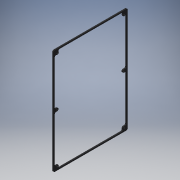
# Autodesk Inventor part: gasket
Saved by Autodesk Inventor 2019 (Build 230136000, 136)
## iProperties
Created: 2020-02-21
Part Number: gasket
Material: Generic
Document SubType Name: Modeling
Designer: ntb11189
Density: 1 g/cm^3
Appearance: Rubber - Black
Author: ntb11189
Autodesk Inventor part; units mm, degrees
ref_plane "YZ Plane" through (0, 0, 0) normal (1, 0, 0) x (0, 1, 0)
ref_plane "XZ Plane" through (0, 0, 0) normal (0, 1, 0) x (-1, 0, 0)
ref_plane "XY Plane" through (0, 0, 0) normal (0, 0, 1) x (1, 0, 0)
sketch "Sketch1" plane through (0, 0, 0) normal (1, 0, 0) x (0, 1, 0)
  line L0 (-4.25, -58.4) -> (-75.9, -58.4)
  arc A0 (-78.2159, -55.4407) -> (-75.9, -58.4) centre (-75.9, -56.0141) ccw
  arc A1 (-78.2159, -55.4407) -> (-80.9407, -52.7159) centre (-80.4, -54.9) ccw
  arc A2 (-83.9, -50.4) -> (-80.9407, -52.7159) centre (-81.5141, -50.4) ccw
  line L1 (-83.9, -50.4) -> (-83.9, 50.4)
  arc A3 (-81.3323, 52.0522) -> (-83.9, 50.4) centre (-82.0846, 50.4) ccw
  arc A4 (-81.3323, 52.0522) -> (-78.2997, 54.9071) centre (-80.4, 54.1) ccw
  arc A5 (-75.9, 58.4) -> (-78.2997, 54.9071) centre (-75.9, 55.8292) ccw
  line L2 (-75.9, 58.4) -> (-4.25, 58.4)
  arc A6 (-2.25, 56.4) -> (-4.25, 58.4) centre (-4.25, 56.4) ccw
  line L3 (-2.25, 56.4) -> (-2.25, 54.5)
  arc A7 (-2.25, 54.5) -> (2.25, 54.5) centre (0, 54.5) ccw
  line L4 (2.25, 54.5) -> (2.25, 56.4)
  arc A8 (4.25, 58.4) -> (2.25, 56.4) centre (4.25, 56.4) ccw
  line L5 (4.25, 58.4) -> (75.9, 58.4)
  arc A9 (77.6729, 55.2614) -> (75.9, 58.4) centre (75.9, 56.33) ccw
  arc A10 (77.6729, 55.2614) -> (80.7614, 52.1729) centre (79.6, 54.1) ccw
  arc A11 (83.9, 50.4) -> (80.7614, 52.1729) centre (81.83, 50.4) ccw
  line L6 (83.9, 50.4) -> (83.9, -50.4)
  arc A12 (80.4071, -52.7997) -> (83.9, -50.4) centre (81.3292, -50.4) ccw
  arc A13 (80.4071, -52.7997) -> (77.5522, -55.8323) centre (79.6, -54.9) ccw
  arc A14 (75.9, -58.4) -> (77.5522, -55.8323) centre (75.9, -56.5846) ccw
  line L7 (75.9, -58.4) -> (4.25, -58.4)
  arc A15 (2.25, -56.4) -> (4.25, -58.4) centre (4.25, -56.4) ccw
  line L8 (2.25, -56.4) -> (2.25, -54.5)
  arc A16 (2.25, -54.5) -> (-2.25, -54.5) centre (0, -54.5) ccw
  line L9 (-2.25, -54.5) -> (-2.25, -56.4)
  arc A17 (-4.25, -58.4) -> (-2.25, -56.4) centre (-4.25, -56.4) ccw
  circle A18 centre (-80.4, -54.9) radius 1.25
  circle A19 centre (-80.4, 54.1) radius 1.25
  circle A20 centre (0, -54.5) radius 1.25
  circle A21 centre (79.6, -54.9) radius 1.25
  circle A22 centre (0, 54.5) radius 1.25
  circle A23 centre (79.6, 54.1) radius 1.25
  arc A24 (-85.9, -58.4) -> (-83.9, -60.4) centre (-83.9, -58.4) ccw
  line L10 (-83.9, -60.4) -> (83.9, -60.4)
  arc A25 (83.9, -60.4) -> (85.9, -58.4) centre (83.9, -58.4) ccw
  line L11 (85.9, -58.4) -> (85.9, 58.4)
  arc A26 (85.9, 58.4) -> (83.9, 60.4) centre (83.9, 58.4) ccw
  line L12 (83.9, 60.4) -> (-83.9, 60.4)
  arc A27 (-83.9, 60.4) -> (-85.9, 58.4) centre (-83.9, 58.4) ccw
  line L13 (-85.9, 58.4) -> (-85.9, -58.4)
  point P0 (0, 0)
  point P1 (0, 0)
  constraints: 44 point on circle, 28 centre point, 28 end point
extrude "Extrusion1" add sketch "Sketch1" along normal blind 2
body "Solid1"
